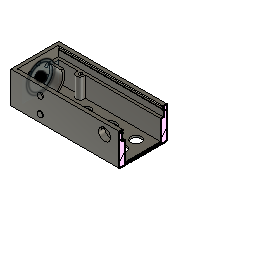
AmpelCase (Autodesk Fusion 360 archive; units mm, degrees)
design "Ampel"
Autodesk Fusion 360 part; units mm, degrees
note: some values were not read from the file. Chosen so that the rebuilt part matches the saved one: which face or edge a step refers to; where a step starts. Set by a fixed rule: which sketch regions a step uses.
sketch "Skizze1" plane through (0, 0, 0) normal (0, 0, 1) x (1, 0, 0)
  line L0 (0, 0) -> (80, 0)
  line L1 (80, 0) -> (80, 20)
  line L2 (80, 20) -> (0, 20)
  line L3 (0, 20) -> (0, 0)
  circle A0 centre (2.5, 2.3) radius 1
  circle A1 centre (78.5, 2.3) radius 1
  circle A2 centre (2.5, 18.3) radius 1
  circle A3 centre (78.5, 18.3) radius 1
  circle A4 centre (6, 3.6) radius 0.5
  circle A5 centre (8.54, 3.6) radius 0.5
  circle A6 centre (11.08, 3.6) radius 0.5
  circle A7 centre (13.62, 3.6) radius 0.5
  circle A8 centre (16.16, 3.6) radius 0.5
  circle A9 centre (18.7, 3.6) radius 0.5
  circle A10 centre (21.24, 3.6) radius 0.5
  circle A11 centre (23.78, 3.6) radius 0.5
  circle A12 centre (26.32, 3.6) radius 0.5
  circle A13 centre (28.86, 3.6) radius 0.5
  circle A14 centre (31.4, 3.6) radius 0.5
  circle A15 centre (33.94, 3.6) radius 0.5
  circle A16 centre (36.48, 3.6) radius 0.5
  circle A17 centre (39.02, 3.6) radius 0.5
  circle A18 centre (41.56, 3.6) radius 0.5
  circle A19 centre (44.1, 3.6) radius 0.5
  circle A20 centre (46.64, 3.6) radius 0.5
  circle A21 centre (49.18, 3.6) radius 0.5
  circle A22 centre (51.72, 3.6) radius 0.5
  circle A23 centre (54.26, 3.6) radius 0.5
  circle A24 centre (56.8, 3.6) radius 0.5
  circle A25 centre (59.34, 3.6) radius 0.5
  circle A26 centre (61.88, 3.6) radius 0.5
  circle A27 centre (64.42, 3.6) radius 0.5
  circle A28 centre (66.96, 3.6) radius 0.5
  circle A29 centre (69.5, 3.6) radius 0.5
  circle A30 centre (72.04, 3.6) radius 0.5
  circle A31 centre (74.58, 3.6) radius 0.5
  circle A32 centre (6, 6.14) radius 0.5
  circle A33 centre (8.54, 6.14) radius 0.5
  circle A34 centre (11.08, 6.14) radius 0.5
  circle A35 centre (13.62, 6.14) radius 0.5
  circle A36 centre (16.16, 6.14) radius 0.5
  circle A37 centre (18.7, 6.14) radius 0.5
  circle A38 centre (21.24, 6.14) radius 0.5
  circle A39 centre (23.78, 6.14) radius 0.5
  circle A40 centre (26.32, 6.14) radius 0.5
  circle A41 centre (28.86, 6.14) radius 0.5
  circle A42 centre (31.4, 6.14) radius 0.5
  circle A43 centre (33.94, 6.14) radius 0.5
  circle A44 centre (36.48, 6.14) radius 0.5
  circle A45 centre (39.02, 6.14) radius 0.5
  circle A46 centre (41.56, 6.14) radius 0.5
  circle A47 centre (44.1, 6.14) radius 0.5
  circle A48 centre (46.64, 6.14) radius 0.5
  circle A49 centre (49.18, 6.14) radius 0.5
  circle A50 centre (51.72, 6.14) radius 0.5
  circle A51 centre (54.26, 6.14) radius 0.5
  circle A52 centre (56.8, 6.14) radius 0.5
  circle A53 centre (59.34, 6.14) radius 0.5
  circle A54 centre (61.88, 6.14) radius 0.5
  circle A55 centre (64.42, 6.14) radius 0.5
  circle A56 centre (66.96, 6.14) radius 0.5
  circle A57 centre (69.5, 6.14) radius 0.5
  circle A58 centre (72.04, 6.14) radius 0.5
  circle A59 centre (74.58, 6.14) radius 0.5
  circle A60 centre (6, 8.68) radius 0.5
  circle A61 centre (8.54, 8.68) radius 0.5
  circle A62 centre (11.08, 8.68) radius 0.5
  circle A63 centre (13.62, 8.68) radius 0.5
  circle A64 centre (16.16, 8.68) radius 0.5
  circle A65 centre (18.7, 8.68) radius 0.5
  circle A66 centre (21.24, 8.68) radius 0.5
  circle A67 centre (23.78, 8.68) radius 0.5
  circle A68 centre (26.32, 8.68) radius 0.5
  circle A69 centre (28.86, 8.68) radius 0.5
  circle A70 centre (31.4, 8.68) radius 0.5
  circle A71 centre (33.94, 8.68) radius 0.5
  circle A72 centre (36.48, 8.68) radius 0.5
  circle A73 centre (39.02, 8.68) radius 0.5
  circle A74 centre (41.56, 8.68) radius 0.5
  circle A75 centre (44.1, 8.68) radius 0.5
  circle A76 centre (46.64, 8.68) radius 0.5
  circle A77 centre (49.18, 8.68) radius 0.5
  circle A78 centre (51.72, 8.68) radius 0.5
  circle A79 centre (54.26, 8.68) radius 0.5
  circle A80 centre (56.8, 8.68) radius 0.5
  circle A81 centre (59.34, 8.68) radius 0.5
  circle A82 centre (61.88, 8.68) radius 0.5
  circle A83 centre (64.42, 8.68) radius 0.5
  circle A84 centre (66.96, 8.68) radius 0.5
  circle A85 centre (69.5, 8.68) radius 0.5
  circle A86 centre (72.04, 8.68) radius 0.5
  circle A87 centre (74.58, 8.68) radius 0.5
  circle A88 centre (6, 11.22) radius 0.5
  circle A89 centre (8.54, 11.22) radius 0.5
  circle A90 centre (11.08, 11.22) radius 0.5
  circle A91 centre (13.62, 11.22) radius 0.5
  circle A92 centre (16.16, 11.22) radius 0.5
  circle A93 centre (18.7, 11.22) radius 0.5
  circle A94 centre (21.24, 11.22) radius 0.5
  circle A95 centre (23.78, 11.22) radius 0.5
  circle A96 centre (26.32, 11.22) radius 0.5
  circle A97 centre (28.86, 11.22) radius 0.5
  circle A98 centre (31.4, 11.22) radius 0.5
  circle A99 centre (33.94, 11.22) radius 0.5
  circle A100 centre (36.48, 11.22) radius 0.5
  circle A101 centre (39.02, 11.22) radius 0.5
  circle A102 centre (41.56, 11.22) radius 0.5
  circle A103 centre (44.1, 11.22) radius 0.5
  circle A104 centre (46.64, 11.22) radius 0.5
  circle A105 centre (49.18, 11.22) radius 0.5
  circle A106 centre (51.72, 11.22) radius 0.5
  circle A107 centre (54.26, 11.22) radius 0.5
  circle A108 centre (56.8, 11.22) radius 0.5
  circle A109 centre (59.34, 11.22) radius 0.5
  circle A110 centre (61.88, 11.22) radius 0.5
  circle A111 centre (64.42, 11.22) radius 0.5
  circle A112 centre (66.96, 11.22) radius 0.5
  circle A113 centre (69.5, 11.22) radius 0.5
  circle A114 centre (72.04, 11.22) radius 0.5
  circle A115 centre (74.58, 11.22) radius 0.5
  circle A116 centre (6, 13.76) radius 0.5
  circle A117 centre (8.54, 13.76) radius 0.5
  circle A118 centre (11.08, 13.76) radius 0.5
  circle A119 centre (13.62, 13.76) radius 0.5
  circle A120 centre (16.16, 13.76) radius 0.5
  circle A121 centre (18.7, 13.76) radius 0.5
  circle A122 centre (21.24, 13.76) radius 0.5
  circle A123 centre (23.78, 13.76) radius 0.5
  circle A124 centre (26.32, 13.76) radius 0.5
  circle A125 centre (28.86, 13.76) radius 0.5
  circle A126 centre (31.4, 13.76) radius 0.5
  circle A127 centre (33.94, 13.76) radius 0.5
  circle A128 centre (36.48, 13.76) radius 0.5
  circle A129 centre (39.02, 13.76) radius 0.5
  circle A130 centre (41.56, 13.76) radius 0.5
  circle A131 centre (44.1, 13.76) radius 0.5
  circle A132 centre (46.64, 13.76) radius 0.5
  circle A133 centre (49.18, 13.76) radius 0.5
  circle A134 centre (51.72, 13.76) radius 0.5
  circle A135 centre (54.26, 13.76) radius 0.5
  circle A136 centre (56.8, 13.76) radius 0.5
  circle A137 centre (59.34, 13.76) radius 0.5
  circle A138 centre (61.88, 13.76) radius 0.5
  circle A139 centre (64.42, 13.76) radius 0.5
  circle A140 centre (66.96, 13.76) radius 0.5
  circle A141 centre (69.5, 13.76) radius 0.5
  circle A142 centre (72.04, 13.76) radius 0.5
  circle A143 centre (74.58, 13.76) radius 0.5
  circle A144 centre (6, 16.3) radius 0.5
  circle A145 centre (8.54, 16.3) radius 0.5
  circle A146 centre (11.08, 16.3) radius 0.5
  circle A147 centre (13.62, 16.3) radius 0.5
  circle A148 centre (16.16, 16.3) radius 0.5
  circle A149 centre (18.7, 16.3) radius 0.5
  circle A150 centre (21.24, 16.3) radius 0.5
  circle A151 centre (23.78, 16.3) radius 0.5
  circle A152 centre (26.32, 16.3) radius 0.5
  circle A153 centre (28.86, 16.3) radius 0.5
  circle A154 centre (31.4, 16.3) radius 0.5
  circle A155 centre (33.94, 16.3) radius 0.5
  circle A156 centre (36.48, 16.3) radius 0.5
  circle A157 centre (39.02, 16.3) radius 0.5
  circle A158 centre (41.56, 16.3) radius 0.5
  circle A159 centre (44.1, 16.3) radius 0.5
  circle A160 centre (46.64, 16.3) radius 0.5
  circle A161 centre (49.18, 16.3) radius 0.5
  circle A162 centre (51.72, 16.3) radius 0.5
  circle A163 centre (54.26, 16.3) radius 0.5
  circle A164 centre (56.8, 16.3) radius 0.5
  circle A165 centre (59.34, 16.3) radius 0.5
  circle A166 centre (61.88, 16.3) radius 0.5
  circle A167 centre (64.42, 16.3) radius 0.5
  circle A168 centre (66.96, 16.3) radius 0.5
  circle A169 centre (69.5, 16.3) radius 0.5
  circle A170 centre (72.04, 16.3) radius 0.5
  circle A171 centre (74.58, 16.3) radius 0.5
  dimension "d1" = 80
  dimension "d2" = 20
  dimension "d3" = 2
  dimension "d6" = 76
  dimension "d7" = 16
  dimension "d8" = 2.3
  dimension "d9" = 2.5
  dimension "d10" = 1
  dimension "d13" = 2.54
  dimension "d14" = 2.54
  dimension "d15" = 3.6
  dimension "d16" = 6
  constraint horizontal L0
  constraint vertical L1
  constraint horizontal L2
  constraint vertical L3
  constraint coincident L0.start L3.end
  measures "d1" distance of L0.start L0.end
  measures "d2" distance of L0.start L2.end
  measures "d3" diameter of A0
  measures "d8" distance of L0 A0.centre
  measures "d9" distance of L3 A0.centre
  measures "d10" diameter of A4
  measures "d15" distance of L0 A4.centre
  measures "d16" distance of L3 A4.centre
extrude "Extrusion1" add sketch "Skizze1" along normal blind 1.5 makes body 1
sketch "Skizze2" plane through (0, 0, 1.5) normal (0, 0, 1) x (-1, 0, 0)
  circle A0 centre (-59.34, -6.14) radius 0.5
  circle A1 centre (-61.88, -6.14) radius 0.5
  circle A2 centre (-36.48, -13.76) radius 0.5
  circle A3 centre (-33.94, -13.76) radius 0.5
  circle A4 centre (-23.78, -13.76) radius 0.5
  circle A5 centre (-21.24, -13.76) radius 0.5
  circle A6 centre (-11.08, -13.76) radius 0.5
  circle A7 centre (-8.54, -13.76) radius 0.5
  circle A8 centre (-46.64, -13.76) radius 0.5
  circle A9 centre (-49.18, -13.76) radius 0.5
  circle A10 centre (-59.34, -13.76) radius 0.5
  circle A11 centre (-61.88, -13.76) radius 0.5
  circle A12 centre (-2.5, -2.3) radius 1
  circle A13 centre (-78.5, -2.3) radius 1
  circle A14 centre (-2.5, -18.3) radius 1
  circle A15 centre (-78.5, -18.3) radius 1
  circle A16 centre (-8.54, -6.14) radius 0.5
  circle A17 centre (-11.08, -6.14) radius 0.5
  circle A18 centre (-21.24, -6.14) radius 0.5
  circle A19 centre (-23.78, -6.14) radius 0.5
  circle A20 centre (-33.94, -6.14) radius 0.5
  circle A21 centre (-36.48, -6.14) radius 0.5
  circle A22 centre (-49.18, -6.14) radius 0.5
  circle A23 centre (-46.64, -6.14) radius 0.5
  line L0 (0, 0) -> (-80, 0)
  line L1 (-80, 0) -> (-80, -20)
  line L2 (0, -20) -> (0, 0)
  line L3 (-80, -20) -> (0, -20)
  circle A24 centre (-2.5, -18.3) radius 1
  circle A25 centre (-2.5, -2.3) radius 1
  circle A26 centre (-78.5, -2.3) radius 1
  circle A27 centre (-78.5, -18.3) radius 1
  circle A28 centre (-9.6934, -13.76) radius 2.625
  circle A29 centre (-22.3934, -13.76) radius 2.625
  circle A30 centre (-35.0934, -13.76) radius 2.625
  circle A31 centre (-47.7934, -13.76) radius 2.625
  circle A32 centre (-60.4934, -13.76) radius 2.625
  circle A33 centre (-9.6934, -6.14) radius 2.625
  circle A34 centre (-22.3934, -6.14) radius 2.625
  circle A35 centre (-35.0934, -6.14) radius 2.625
  circle A36 centre (-47.7934, -6.14) radius 2.625
  circle A37 centre (-60.4934, -6.14) radius 2.625
  line L4 (-80, 0) -> (10, 0)
  line L5 (10, 0) -> (10, -20)
  line L6 (10, -20) -> (-80, -20)
  line L7 (-80, -20) -> (-80, 0)
  line L8 (10.4, -20.4) -> (-80.4, -20.4)
  line L9 (-80.4, -20.4) -> (-80.4, 0.4)
  line L10 (-80.4, 0.4) -> (10.4, 0.4)
  line L11 (10.4, 0.4) -> (10.4, -20.4)
  line L12 (9, -19) -> (-79, -19)
  line L13 (-79, -19) -> (-79, -1)
  line L14 (-79, -1) -> (9, -1)
  line L15 (9, -1) -> (9, -19)
  line L16 (12, -22) -> (-82, -22)
  line L17 (-82, -22) -> (-82, 2)
  line L18 (-82, 2) -> (12, 2)
  line L19 (12, 2) -> (12, -22)
  circle A38 centre (-78.5, -18.3) radius 2
  circle A39 centre (-78.5, -2.3) radius 2
  circle A40 centre (-2.5, -18.3) radius 2
  circle A41 centre (-2.5, -2.3) radius 2
  circle A42 centre (-2.5, -2.3) radius 0.8
  circle A43 centre (-2.5, -18.3) radius 0.8
  circle A44 centre (-78.5, -18.3) radius 0.8
  circle A45 centre (-78.5, -2.3) radius 0.8
  dimension "d19" = 5.25
  dimension "d22" = -12.7
  dimension "d23" = 7.62
  dimension "d39" = 90
  dimension "d40" = 19.5066
  dimension "d41" = 19.6934
  dimension "d42" = -0.4
  dimension "d43" = 1
  dimension "d44" = -2
  dimension "d51" = 1
  dimension "d52" = 1
  dimension "d53" = 1
  dimension "d54" = 1
  dimension "d55" = -0.2
  dimension "d56" = -0.2
  dimension "d57" = -0.2
  dimension "d58" = -0.2
  dimension "d126" = 5.25
  constraint horizontal L4
  constraint vertical L5
  constraint horizontal L6
  constraint vertical L7
  constraint coincident L0.end L1.start
  measures "d19" diameter of A28
  measures "d39" distance of L0.end L4.end
  measures "d40" distance of A37.centre L7
  measures "d41" distance of A33.centre L5
  measures "d51" distance of A15
  measures "d52" distance of A13
  measures "d53" distance of A14
  measures "d54" distance of A12
  measures "d126" diameter of A29
extrude "Extrusion6" add sketch "Skizze2" along normal blind 10 separate body contours A13 A26 L13 A45 | A13 L1 A26 L7 L13 L14 A39 | L13 A45 | L1 L7 L13 A38 A39 | L0 L1 L2 L4 L7 L14 A39 A41 | A15 L1 L3 A27 L6 L7 L12 L13 A38 | L1 L7 L9 A39 | L1 L7 L9 A38 A39 | L14 A41 | L0 L1 L3 L4 L5 L6 L7 L8 L9 L10 L11 A38 A39 A40 | A15 A27 L12 L13 A44 | L1 L7 L9 A38 | L13 A44 | L3 L6 L12 A38 A40 | L1 L3 L6 L7 A38 | L2 L4 L5 L6 L12 L14 L15 | L12 A44 | A14 L3 A24 L6 L12 A40 | L3 L6 A38 | L2 L3 L6 L12 A40 | L3 L6 A40 picked at (-79.1188, -2.9955) picked at (-79.1077, -2.5082) picked at (-2.4352, -0.5332) picked at (-78.9279, -19.1273) makes body 2
extrude "Extrusion7" add sketch "Skizze2" along normal up to surface (15 mm away) contours L9 A39 | L9 A38 | L16 L17 L18 L19 bodies 2
extrude "Extrusion8" add sketch "Skizze2" against normal blind 1 contours A12 A25 | A13 A26 L13 A45 | A13 A26 L13 L14 A39 | A13 A26 L13 A45 | A13 L1 A26 L7 L13 L14 A39 | L13 A45 | L13 A45 | L2 L12 L13 L14 A38 A39 A40 A41 | L1 L7 L13 A38 A39 | L0 L1 L2 L4 L7 L14 A39 A41 | A15 A27 L12 L13 A38 | A15 L1 L3 A27 L6 L7 L12 L13 A38 | L1 L7 L9 A39 | L1 L7 L9 A38 A39 | L14 A41 | L14 A41 | L0 L1 L3 L4 L5 L6 L7 L8 L9 L10 L11 A38 A39 A40 | A15 A27 L12 L13 A44 | A15 A27 L12 L13 A44 | L1 L7 L9 A38 | L9 A39 | L12 L13 A44 | L13 A44 | L3 L6 L12 A38 A40 | L1 L3 L6 L7 A38 | L9 A38 | L2 L12 L14 L15 | L2 L4 L5 L6 L12 L14 L15 | L12 A44 | L12 L13 A44 | A14 A24 L12 A40 | A14 L3 A24 L6 L12 A40 | L3 L6 A38 | L2 L3 L6 L12 A40 | A14 A24 L12 A43 | A14 A24 L12 A43 | L3 L6 A40 | L12 A43 | L12 A43 | L16 L17 L18 L19 | A42 bodies 2
extrude "Extrusion9" add sketch "Skizze2" along normal up to surface (10 mm away) contours A12 A25 | A13 A26 L13 A45 | A13 A26 L13 L14 A39 | A15 A27 L12 L13 A38 | L14 A41 | A15 A27 L12 L13 A44 | A14 A24 L12 A40 | A14 A24 L12 A43 picked at (-78.8863, -3.147) picked at (-2.5249, -1.1009) picked at (-78.8863, -17.453) picked at (-3.1978, -18.9164) bodies 2
extrude "Extrusion10" cut sketch "Skizze2" along normal up to surface (10 mm away) contours L13 A45 | L13 A45 | L12 L13 A44 | L13 A44 | L12 A44 picked at (-78.4962, -18.3026) bodies 2
sketch "Skizze3" plane through (82, 0, 0) normal (1, 0, 0) x (0, 1, 0)
  line L0 (22, 16.5) -> (-2, 16.5)
  line L1 (-2, 16.5) -> (-2, 0.5)
  line L2 (-2, 0.5) -> (22, 0.5)
  line L3 (22, 0.5) -> (22, 16.5)
  line L4 (-23.7892, 8.5) -> (19.7892, 8.5) construction
  circle A0 centre (-14, 8.5) radius 8.15
  circle A1 centre (-14, 8.5) radius 9.65
  line L5 (-14, 8.5) -> (-14, 21.0913) construction
  line L6 (-12.6056, 18.0487) -> (-2, 16.5)
  line L7 (-12.6056, -1.0487) -> (-2, 0.5)
  dimension "d64" = 16.3
  dimension "d65" = 1.5
  dimension "d66" = 12
  constraint horizontal L4
  constraint midpoint L1 L4
  constraint coincident L4 A0.centre
  constraint coincident A0.centre A1.centre
  constraint perpendicular L4 L5
  constraint coincident L0.end L1.start
  constraint tangent A1 L6
  constraint coincident A1 L6.start
  constraint symmetric L4 L0.end L1.end
  constraint symmetric L4 L6.start L7.start
  measures "d64" diameter of A0
  measures "d66" distance of L1 A0.centre
extrude "Extrusion11" add sketch "Skizze3" against normal blind 10 from surface at -10 contours L1 A1 L6 L7 | A1 bodies 2
extrude "Extrusion12" add sketch "Skizze3" along normal blind 10 from surface at -84 contours L1 A1 L6 L7 | A1 bodies 2
sketch "Skizze4" plane through (0, -2, 0) normal (0, -1, 0) x (1, 0, 0)
  line L0 (8, 16.5) -> (8, 0.5)
  line L1 (8, 0.5) -> (62, 0.5)
  line L2 (62, 0.5) -> (62, 16.5)
  line L3 (62, 16.5) -> (8, 16.5)
  line L4 (8, 16.5) -> (62, 0.5) construction
  line L5 (62, 16.5) -> (8, 0.5) construction
  circle A0 centre (35, 11.6289) radius 3
  dimension "d73" = 3
  constraint coincident L0.start L3.end
  constraint coincident L1.end L2.start
  constraint coincident L2.end L3.start
  constraint coincident L0.end L1.start
  constraint tangent L4 A0
  constraint tangent L5 A0
  measures "d73" radius of A0
extrude "Extrusion13" cut sketch "Skizze4" against normal up to surface (3 mm away) contours A0 bodies 2
sketch "Skizze5" plane through (-12, 0, 0) normal (-1, 0, 0) x (0, -1, 0)
  line L0 (2, 16.5) -> (-22, 16.5)
  line L1 (-22, 16.5) -> (-22, 0.5)
  line L2 (-22, 0.5) -> (2, 0.5)
  line L3 (2, 0.5) -> (2, 16.5)
  line L4 (-22, 16.5) -> (2, 0.5) construction
  line L5 (2, 16.5) -> (-22, 0.5) construction
  circle A0 centre (-10, 8.5) radius 5 construction
  circle A1 centre (-5.8397, 11.2735) radius 1
  circle A2 centre (-10.3218, 13.4896) radius 1
  circle A3 centre (-14.482, 10.7161) radius 1
  circle A4 centre (-14.1603, 5.7265) radius 1
  circle A5 centre (-9.6782, 3.5104) radius 1
  circle A6 centre (-5.518, 6.2839) radius 1
  circle A7 centre (-10, 8.5) radius 1
  dimension "d79" = 10
  dimension "d80" = 2
  dimension "d82" = 360
  dimension "d83" = 2
  constraint coincident L0.end L1.start
  constraint coincident L2.end L3.start
  constraint coincident L0.start L3.end
  constraint coincident L1.end L2.start
  constraint midpoint L5 A0.centre
  constraint coincident A0 A1.centre
  constraint coincident L5 A1.centre
  constraint concentric A0 A7
  measures "d79" diameter of A0
  measures "d80" diameter of A1
  measures "d83" diameter of A7
extrude "Extrusion14" cut sketch "Skizze5" against normal up to surface (3 mm away) contours A1 | A2 | A3 | A4 | A5 | A6 | A7 bodies 2
sketch "Skizze6" plane through (82, 0, 0) normal (1, 0, 0) x (0, 1, 0)
  line L0 (22, 16.5) -> (-2, 16.5)
  line L1 (-2, 16.5) -> (-2, 0.5)
  line L2 (-2, 0.5) -> (22, 0.5)
  line L3 (22, 0.5) -> (22, 16.5)
  line L4 (10, 19.0897) -> (10, 13.1499) construction
  line L5 (21, 15) -> (-1, 15)
  line L6 (-1, 15) -> (-1, 18)
  line L7 (-1, 18) -> (21, 18)
  line L8 (21, 18) -> (21, 15)
  line L9 (21, 15) -> (-1, 18) construction
  line L10 (-1, 15) -> (21, 18) construction
  line L11 (-2, 16.5) -> (-2, 0.5)
  line L12 (-1, 15) -> (4, 23.6603)
  line L13 (-1, 15) -> (9.5, 15) construction
  line L14 (21, 15) -> (16, 23.6603)
  line L15 (-1, 15) -> (-0.2, 15)
  line L16 (-1, 15) -> (-1, 13)
  line L17 (-1, 13) -> (-0.2, 15)
  line L18 (21, 15) -> (20.2, 15)
  line L19 (21, 15) -> (21, 13)
  line L20 (21, 13) -> (20.2, 15)
  point P0 (10, 16.5)
  point P1 (22, 16.5)
  dimension "d86" = 3
  dimension "d87" = 1
  dimension "d88" = 1
  dimension "d89" = 60
  dimension "d90" = 10
  dimension "d91" = 10
  dimension "d92" = 60
  dimension "d97" = 0.8
  dimension "d98" = 2
  constraint vertical L4
  constraint horizontal L5
  constraint perpendicular L5 L6
  constraint parallel L5 L7
  constraint parallel L6 L8
  constraint coincident L9 P0
  constraint coincident L10 P0
  constraint coincident L0 P0
  constraint coincident L4 P0
  constraint horizontal L13
  constraint perpendicular L6 L15
  constraint perpendicular L15 L16
  constraint symmetric L4 L5.end L5.start
  constraint symmetric L4 L15.end L18.end
  constraint symmetric L4 L16.end L19.end
  measures "d86" distance of L5.end L6.end
  measures "d87" distance of L6 L11
  measures "d88" distance of L8 P1
  measures "d89" angle of L12 L13
  measures "d90" distance of L5.end L12.end
  measures "d91" distance of L5.start L14.end
  measures "d92" angle of L5 L14
  measures "d97" distance of L5.end L15.end
  measures "d98" distance of L5.end L16.end
extrude "Extrusion15" cut sketch "Skizze6" against normal up to surface (92.4 mm away) contours L0 L5 L12 L14 L15 L18 bodies 2
extrude "Extrusion16" add sketch "Skizze6" against normal up to surface (92.4 mm away) contours L0 L8 L14 | L0 L6 L12 bodies 2
extrude "Extrusion17" add sketch "Skizze6" against normal up to surface (92.4 mm away) contours L5 L18 L19 L20 | L5 L15 L16 L17 bodies 2
extrude "Extrusion18" cut sketch "Skizze4" against normal up to surface (21 mm away) contours A0 bodies 2
extrude "Extrusion19" add sketch "Skizze6" against normal up to surface (92.4 mm away) separate body contours L0 L5 L12 L14 L15 L18 makes body 3
scale "Maßstab1" factors (1, 1, 0.98) about (-10.4, -0.134, 16.5) bodies 3
split "Teilen1" by plane through (82, -2, 1.5) normal (0, -1, 0) bodies 2 makes body 4 at (4.6667, -5.8601, 8.0938) makes body 5 at (65.3333, -5.8601, 8.0938)
sketch "Skizze7" plane through (0, -2, 0) normal (0, 1, 0) x (-1, 0, 0)
  line L0 (-72, 0.5) -> (-62, 0.5)
  line L1 (-62, 0.5) -> (-62, 16.5)
  line L2 (-62, 16.5) -> (-72, 16.5)
  line L3 (-72, 16.5) -> (-72, 0.5)
  line L4 (-8, 16.5) -> (-8, 0.5)
  line L5 (-8, 0.5) -> (2, 0.5)
  line L6 (2, 0.5) -> (2, 16.5)
  line L7 (2, 16.5) -> (-8, 16.5)
  line L8 (-67, 37.408) -> (-67, -4.408) construction
  line L9 (-3, 43.7015) -> (-3, -10.7015) construction
  line L10 (-75.2755, 12.5) -> (5.161, 12.5) construction
  line L11 (-75.2755, 4.5) -> (5.161, 4.5) construction
  circle A0 centre (-67, 12.5) radius 1.5
  circle A1 centre (-67, 4.5) radius 1.5
  circle A2 centre (-3, 12.5) radius 1.5
  circle A3 centre (-3, 4.5) radius 1.5
  dimension "d108" = 16
  dimension "d109" = 4
  dimension "d110" = 4
  dimension "d111" = 3
  dimension "d112" = 3
  dimension "d113" = 3
  dimension "d114" = 3
  constraint vertical L8
  constraint midpoint L2 L8
  constraint parallel L6 L9
  constraint midpoint L7 L9
  constraint perpendicular L6 L10
  constraint parallel L10 L11
  constraint coincident L8 A0.centre
  constraint coincident L10 A0.centre
  constraint coincident L8 A1.centre
  constraint coincident L11 A1.centre
  constraint coincident L9 A2.centre
  constraint coincident L10 A2.centre
  constraint coincident L11 A3.centre
  constraint coincident L9 A3.centre
  measures "d108" distance of L0.end L1.end
  measures "d109" distance of L2 L10
  measures "d110" distance of L0 L11
  measures "d111" diameter of A0
  measures "d112" diameter of A1
  measures "d113" diameter of A2
  measures "d114" diameter of A3
extrude "Extrusion20" cut sketch "Skizze7" against normal blind 0.5 contours A0 | A1 | A2 | A3 bodies 4 5
extrude "Extrusion21" add sketch "Skizze7" against normal blind 0.5 contours A0 | A1 | A2 | A3 bodies 2
move_face "Flächen versetzen1" offset -0.15 4 faces at (1.5075, -2.1667, 12.3506) (1.5075, -2.1667, 4.3506) (66.5937, -2.3333, 5.9439) (66.5937, -2.3333, 13.9439) on bodies 2
sketch "Skizze9" plane through (-9, 0, 0) normal (1, 0, 0) x (0, 1, 0)
  arc A0 (13.8611, 11.5) -> (15.103, 11.5) centre (14.482, 10.7161) ccw
  line L0 (13.8611, 11.5) -> (6.8138, 11.5)
  arc A1 (4.8657, 11.5) -> (6.8138, 11.5) centre (5.8397, 11.2735) ccw
  line L1 (4.8657, 11.5) -> (1, 11.5)
  line L2 (1, 11.5) -> (1, 1.5)
  line L3 (1, 1.5) -> (19, 1.5)
  line L4 (19, 1.5) -> (19, 11.5)
  line L5 (19, 11.5) -> (15.103, 11.5)
  circle A2 centre (5.518, 6.2839) radius 1
  circle A3 centre (10, 8.5) radius 1
  circle A4 centre (9.6782, 3.5104) radius 1
  circle A5 centre (14.1603, 5.7265) radius 1
  circle A6 centre (10, 8.5) radius 6
  circle A7 centre (10, 8.5) radius 7.1
  point P0 (10, 8.5)
  dimension "d122" = 12
  dimension "d123" = 1.1
  constraint coincident P0 A3.centre
  measures "d122" diameter of A6
extrude "Extrusion22" add sketch "Skizze9" along normal blind 5 contours L1 L3 L5 A6 A7 bodies 2
extrude "Extrusion23" cut sketch "Skizze9" against normal up to surface (1.4 mm away) contours A0 L0 A1 L1 L5 A6 | A0 L0 A1 L1 A6 bodies 2
hidden bodies 1 3 4 5
equation "d22 = ( -2.54 * 5 ) * 1 mm"
equation "d23 = ( 2.54 * 3 ) * 1 mm"
equation "d39 = 94 mm - 4 mm"
named bodies: "PCB", "Gehäuse", "Deckel", "Halter1", "Halter2"
